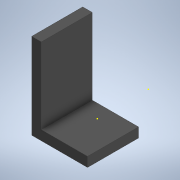
# Autodesk Inventor part: silla aleta
Saved by Autodesk Inventor 2021.2 (Build 252289000, 289)
## iProperties
Created: 2021-04-11
Part Number: silla aleta
Material: Sillas
Document SubType Name: Modeling
Designer: equip
Density: 1.6527 g/cm^3
Appearance: Genérico
Mass: 120003 g
Surface Area: 18322 cm^2
Volume: 72610 cm^3
Author: equip
Autodesk Inventor part; units mm, degrees
ref_plane "YZ Plane" through (0, 0, 0) normal (1, 0, 0) x (0, 1, 0)
ref_plane "XZ Plane" through (0, 0, 0) normal (0, 1, 0) x (-1, 0, 0)
ref_plane "XY Plane" through (0, 0, 0) normal (0, 0, 1) x (1, 0, 0)
sketch "Boceto1" plane through (0, 0, 0) normal (0, 1, 0) x (-1, 0, 0)
  point P0 (0, 0)
sketch "Boceto2" plane through (0, 0, 0) normal (0, 1, 0) x (-1, 0, 0)
  point P0 (0, 0)
sketch "Boceto3" plane through (0, 0, 0) normal (0, 0, 1) x (1, 0, 0)
  line L0 (-681.5559, 400.996) -> (-581.5559, 400.996)
  line L1 (-101.5559, -489.004) -> (-681.5559, -489.004)
  line L2 (-681.5559, -489.004) -> (-681.5559, 400.996)
  line L3 (-101.5559, -489.004) -> (-101.5559, -389.004)
  line L4 (-101.5559, -389.004) -> (-581.5559, -389.004)
  line L5 (-581.5559, -389.004) -> (-581.5559, 400.996)
  point P0 (0, 0)
  dimension "d0" = 580
  dimension "d2" = 100
  dimension "d3" = 480
  constraints: 12 end point, 2 perpendicular, 1 horizontal, 1 parallel
  measures "d0" distance of L1.start L1.end
  measures "d2" distance of L1.start L3.end
  measures "d3" distance of L3.end L4.end
extrude "Extrusión1" add sketch "Boceto3" along normal blind 530
sketch "Boceto4" plane through (0, 0, 530) normal (0, 0, 1) x (1, 0, 0)
  point P0 (0, 0)
